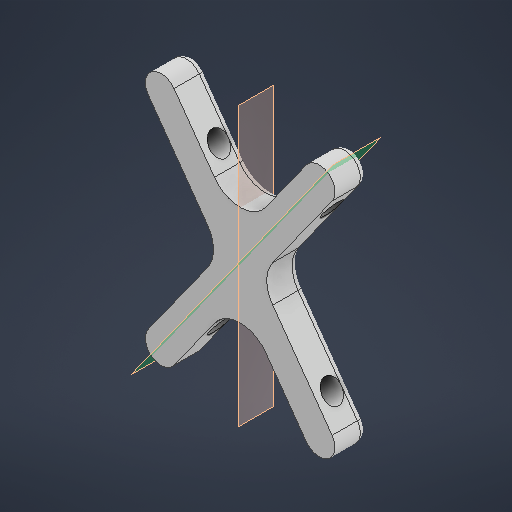
# Autodesk Inventor part: vetrovaniig
Saved by Autodesk Inventor 2026 (Build 300175050, 175E)
## iProperties
Created: 2026-02-22
Part Number: vetrovaniig
Material: Všeobecné
Document SubType Name: Modeling
Designer: marti
Density: 1 g/cm^3
Appearance: Výchozí
Author: marti
Autodesk Inventor part; units mm, degrees
ref_plane "XZ Plane" through (0, 0, 0) normal (0, 1, 0) x (-1, 0, 0)
ref_plane "XY Plane" through (0, 0, 0) normal (0, 0, 1) x (1, 0, 0)
sketch "Náčrt1" plane through (0, 0, 0) normal (0, 0, 1) x (1, 0, 0)
  line L0 (25, -35) -> (-25, 35) construction
  line L1 (-25, -35) -> (25, 35) construction
  arc A0 (-20.9313, 37.9062) -> (-29.0687, 32.0938) centre (-25, 35) ccw
  arc A1 (29.0687, 32.0938) -> (20.9313, 37.9062) centre (25, 35) ccw
  arc A2 (-29.0687, -32.0938) -> (-20.9313, -37.9062) centre (-25, -35) ccw
  arc A3 (20.9313, -37.9062) -> (29.0687, -32.0938) centre (25, -35) ccw
  line L2 (20.9313, 37.9062) -> (0, 8.6023)
  line L3 (-6.1445, 0) -> (-29.0687, -32.0938)
  line L4 (29.0687, -32.0938) -> (6.1445, 0)
  line L5 (0, 8.6023) -> (-20.9313, 37.9062)
  line L6 (-20.9313, -37.9062) -> (0, -8.6023)
  line L7 (6.1445, 0) -> (29.0687, 32.0938)
  line L8 (-29.0687, 32.0938) -> (-6.1445, 0)
  line L9 (0, -8.6023) -> (20.9313, -37.9062)
  line L10 (-44.7648, 0) -> (44.7648, 0) projected
  line L11 (0, 58.7648) -> (0, -58.7648) projected
  point P0 (0, 0)
  dimension "d2" = 50
  dimension "d3" = 70
  dimension "d7" = 10
  dimension "d8" = 10
  dimension "d9" = 10
  dimension "d10" = 10
  dimension "d56" = 71.075
  dimension "d57" = 108.925
  constraints: 20 end point, 12 tangent, 8 point on circle, 4 centre point, 3 coincident, 2 midpoint
  measures "d2" distance of L1.end L0.end
  measures "d3" distance of L0.end L1.start
  measures "d7" diameter of A0
  measures "d8" diameter of A1
  measures "d9" diameter of A2
  measures "d10" diameter of A3
  measures "d56" angle of L5 L2
  measures "d57" angle of L4 L7
extrude "Vysunutí1" add sketch "Náčrt1" along normal mid plane 10
fillet "Zaoblení1" radius 10 4 edges at (6.1445, 0, 0) (-6.1445, 0, 0) (0, 8.6023, 0) (0, -8.6023, 0)
ref_plane "Pracovní rovina4" through (0, 0, 0) normal (1, 0, 0) x (0, 1, 0)
sketch "Náčrt4" plane through (0, 0, 0) normal (1, 0, 0) x (0, 1, 0)
  line L0 (-35, 0) -> (35, 0) projected
  line L1 (0, 35) -> (0, -35) projected
  point P0 (0, 0)
  point P1 (25, 0)
  point P2 (-25, 0)
  constraints: 2 point on line
hole "Díra1" at (0, 25, 0) at (0, -25, 0) direction (-1, 0, 0) diameter 6 end through all both
fillet "Zaoblení3" radius 2 12 edges at (-19.6824, 18.9531, -5) (-27.9062, 39.0687, -5) (-14.5343, 28.9504, -5) (14.5343, 28.9504, -5) (27.9062, 39.0687, -5) (19.6824, 18.9531, -5) (19.6824, -18.9531, -5) (27.9062, -39.0687, -5) (14.5343, -28.9504, -5) (-14.5343, -28.9504, -5) (-27.9062, -39.0687, -5) (-19.6824, -18.9531, -5)
ref_plane "Pracovní rovina5" through (-25, -35, -3) normal (-0.8137, 0.5812, 0) x (0, 0, 1)
